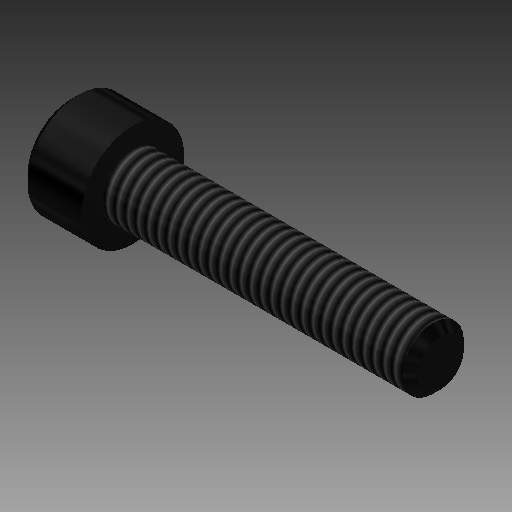
# Autodesk Inventor part: M6x30
Saved by Autodesk Inventor 2019 (Build 230136000, 136)
## iProperties
Created: 2015-07-16
Part Number: M6x30
Material: Stainless Steel
Document SubType Name: Modeling
Designer: yxb10131
Density: 8 g/cm^3
Appearance: Glossy - Black
Description: Plain M6 Bolt
Author: yxb10131
Autodesk Inventor part; units mm, degrees
ref_plane "YZ Plane" through (0, 0, 0) normal (1, 0, 0) x (0, 1, 0)
ref_plane "XZ Plane" through (0, 0, 0) normal (0, 1, 0) x (-1, 0, 0)
ref_plane "XY Plane" through (0, 0, 0) normal (0, 0, 1) x (1, 0, 0)
sketch "Sketch1" plane through (0, 0, 0) normal (0, 0, 1) x (1, 0, 0)
  line L0 (0, 6) -> (0, -1) projected
  line L1 (-7.2, 0) -> (43.2, 0) projected
  line L2 (0, 5) -> (6, 5)
  line L3 (6, 5) -> (6, 3)
  line L4 (6, 3) -> (36, 3)
  line L5 (36, 3) -> (36, 0)
  line L6 (0, 0) -> (36, 0)
  line L7 (0, 5) -> (0, 0)
  dimension "d0" = 30
  dimension "d1" = 10
  dimension "d2" = 6
  dimension "d3" = 6
  constraints: 12 end point, 3 perpendicular, 2 collinear, 2 point on line, 1 horizontal
  measures "d0" distance of L3.end L4.end
  measures "d1" diameter of L2 L1
  measures "d2" diameter of L4 L1
  measures "d3" distance of L2.start L2.end
revolve "Revolution1" add sketch "Sketch1" angle 360 about axis through (0, 0, 0) along (1, 0, 0)
sketch "Sketch2" plane through (0, 0, 0) normal (-1, 0, 0) x (0, 0, 1)
  line L0 (-7, 0) -> (7, 0) projected
  line L1 (0, 7) -> (0, -7) projected
  line L2 (1.4434, -2.5) -> (-1.4434, -2.5)
  line L3 (-1.4434, -2.5) -> (-2.8868, 0)
  line L4 (-2.8868, 0) -> (-1.4434, 2.5)
  line L5 (-1.4434, 2.5) -> (1.4434, 2.5)
  line L6 (1.4434, 2.5) -> (2.8868, 0)
  line L7 (2.8868, 0) -> (1.4434, -2.5)
  point P0 (0, 0)
  point P1 (0, 0)
  dimension "d5" = 5
  constraints: 12 end point, 1 coincident, 1 parallel, 13 other
  measures "d5" distance between parallel lines of L2 L5
extrude "Extrusion1" cut sketch "Sketch2" against normal blind 5
thread "Thread1" size "M6x1" class "6g" standard "ANSI Metric M Profile" full length
chamfer "Chamfer1" distance 0.75 angle 45 2 edges at (0, -5, 0) (36, -3, 0)
body "Solid1"
